Autodesk Fusion 360 part; units mm, degrees
(part 2 of 3)
  spline S292 degree 3 poles (-119.6869, 0.8689) (-119.9271, 0.6416) (-120.1494, 0.602) (-120.3986, 0.874) knots 0 0 0 0 1 1 1 1
  spline S293 degree 3 poles (-120.3986, 0.874) (-120.6491, 1.1474) (-120.9787, 1.2392) (-121.3477, 1.1905) knots 0 0 0 0 1 1 1 1
  spline S294 degree 3 poles (-121.3477, 1.1905) (-121.5549, 1.1631) (-121.713, 1.0742) (-121.7659, 0.8603) knots 0 0 0 0 1 1 1 1
  spline S295 degree 3 poles (-121.7659, 0.8603) (-121.8248, 0.6223) (-121.7241, 0.4521) (-121.5106, 0.3512) knots 0 0 0 0 1 1 1 1
  spline S296 degree 3 poles (-121.5106, 0.3512) (-121.1033, 0.1585) (-120.6785, -0.0017) (-120.2865, -0.221) knots 0 0 0 0 1 1 1 1
  spline S297 degree 3 poles (-120.2865, -0.221) (-119.417, -0.7075) (-119.0197, -1.6781) (-119.281, -2.6156) knots 0 0 0 0 1 1 1 1
  spline S298 degree 3 poles (-119.281, -2.6156) (-119.4987, -3.3967) (-120.0372, -3.8655) (-120.8096, -4.0071) knots 0 0 0 0 1 1 1 1
  spline S299 degree 3 poles (-120.8096, -4.0071) (-121.664, -4.1637) (-122.4734, -4.0633) (-123.0688, -3.3088) knots 0 0 0 0 1 1 1 1
  spline S300 degree 3 poles (-123.0688, -3.3088) (-123.2667, -3.0579) (-123.2642, -2.865) (-123.0212, -2.6394) knots 0 0 0 0 1 1 1 1
  spline S301 degree 3 poles (-123.0212, -2.6394) (-122.4403, -2.1) (-122.3298, -2.0653) (-121.6554, -2.4022) knots 0 0 0 0 1 1 1 1
  spline S302 degree 3 poles (-121.6554, -2.4022) (-121.3441, -2.5577) (-121.0624, -2.5327) (-120.8747, -2.2487) knots 0 0 0 0 1 1 1 1
  spline S303 degree 3 poles (-120.8747, -2.2487) (-120.6748, -1.9465) (-120.8812, -1.7016) (-121.122, -1.5519) knots 0 0 0 0 1 1 1 1
  spline S304 degree 3 poles (-121.122, -1.5519) (-121.3991, -1.3797) (-121.711, -1.259) (-122.0168, -1.1387) knots 0 0 0 0 1 1 1 1
  spline S305 degree 3 poles (-122.0168, -1.1387) (-122.3785, -0.9965) (-122.7031, -0.8076) (-122.9863, -0.484) knots 0 0 0 0 1 1 1 1
  spline S306 degree 3 poles (-129.5748, -3.9986) (-130.0779, -3.6151) (-129.8967, -3.1145) (-129.8126, -2.6894) knots 0 0 0 0 1 1 1 1
  spline S307 degree 3 poles (-129.8126, -2.6894) (-129.7416, -2.3309) (-129.331, -2.397) (-129.0513, -2.4282) knots 0 0 0 0 1 1 1 1
  spline S308 degree 3 poles (-129.0513, -2.4282) (-128.508, -2.4889) (-128.3687, -2.2636) (-128.3813, -1.7476) knots 0 0 0 0 1 1 1 1
  spline S309 degree 3 poles (-128.3813, -1.7476) (-128.4113, -0.5149) (-128.3747, 0.7193) (-128.3882, 1.9526) knots 0 0 0 0 1 1 1 1
  spline S310 degree 3 poles (-128.3882, 1.9526) (-128.3933, 2.4157) (-128.2265, 2.6017) (-127.7479, 2.6027) knots 0 0 0 0 1 1 1 1
  spline S311 degree 3 poles (-127.7479, 2.6027) (-126.5945, 2.6052) (-126.5944, 2.623) (-126.5928, 1.4801) knots 0 0 0 0 1 1 1 1
  spline S312 degree 3 poles (-126.5928, 1.4801) (-126.5912, 0.3682) (-126.5753, -0.7439) (-126.5959, -1.8554) knots 0 0 0 0 1 1 1 1
  spline S313 degree 3 poles (-126.5959, -1.8554) (-126.6037, -2.2776) (-126.4743, -2.4417) (-126.0346, -2.4338) knots 0 0 0 0 1 1 1 1
  spline S314 degree 3 poles (-126.0346, -2.4338) (-125.2421, -2.4195) (-124.8555, -3.1182) (-125.2315, -3.822) knots 0 0 0 0 1 1 1 1
  spline S315 degree 3 poles (-125.2315, -3.822) (-125.3441, -4.0327) (-125.5369, -4.0315) (-125.7256, -4.0311) knots 0 0 0 0 1 1 1 1
  spline S316 degree 3 poles (-125.7256, -4.0311) (-126.9936, -4.028) (-128.2615, -4.0194) (-129.5748, -3.9986) knots 0 0 0 0 1 1 1 1
  spline S317 degree 3 poles (-151.8161, -2.4591) (-151.7724, -2.7435) (-151.9201, -3.0231) (-151.6525, -3.2497) knots 0 0 0 0 1 1 1 1
  spline S318 degree 3 poles (-151.6525, -3.2497) (-151.3521, -3.0403) (-151.5054, -2.7385) (-151.4726, -2.4901) knots 0 0 0 0 1 1 1 1
  spline S319 degree 3 poles (-151.4726, -2.4901) (-151.45, -2.3191) (-151.4678, -2.1432) (-151.4568, -1.9701) knots 0 0 0 0 1 1 1 1
  spline S320 degree 3 poles (-151.4568, -1.9701) (-151.4461, -1.8001) (-151.3237, -1.7311) (-151.1748, -1.7199) knots 0 0 0 0 1 1 1 1
  spline S321 degree 3 poles (-151.1748, -1.7199) (-150.9979, -1.7065) (-150.9253, -1.8309) (-150.9167, -1.9813) knots 0 0 0 0 1 1 1 1
  spline S322 degree 3 poles (-150.9167, -1.9813) (-150.9028, -2.2236) (-150.9108, -2.467) (-150.9054, -2.7099) knots 0 0 0 0 1 1 1 1
  spline S323 degree 3 poles (-150.9054, -2.7099) (-150.8995, -2.9796) (-150.9741, -3.2813) (-150.5847, -3.3799) knots 0 0 0 0 1 1 1 1
  spline S324 degree 3 poles (-150.5847, -3.3799) (-150.4389, -3.4169) (-150.4547, -3.5703) (-150.4745, -3.6907) knots 0 0 0 0 1 1 1 1
  spline S325 degree 3 poles (-150.4745, -3.6907) (-150.4965, -3.8235) (-150.6099, -3.8351) (-150.7149, -3.8355) knots 0 0 0 0 1 1 1 1
  spline S326 degree 3 poles (-150.7149, -3.8355) (-151.2185, -3.8373) (-151.7221, -3.8387) (-152.2257, -3.833) knots 0 0 0 0 1 1 1 1
  spline S327 degree 3 poles (-152.2257, -3.833) (-152.6223, -3.8286) (-152.4677, -3.3848) (-152.687, -3.2345) knots 0 0 0 0 1 1 1 1
  spline S328 degree 3 poles (-152.687, -3.2345) (-152.7158, -3.2563) (-152.7521, -3.2703) (-152.7654, -3.296) knots 0 0 0 0 1 1 1 1
  spline S329 degree 3 poles (-152.7654, -3.296) (-152.8885, -3.5349) (-152.8614, -3.9369) (-153.3119, -3.8241) knots 0 0 0 0 1 1 1 1
  spline S330 degree 3 poles (-153.3119, -3.8241) (-153.728, -3.72) (-153.5082, -3.3696) (-153.5522, -3.1274) knots 0 0 0 0 1 1 1 1
  spline S331 degree 3 poles (-153.5522, -3.1274) (-153.5827, -2.9593) (-153.5583, -2.7811) (-153.5579, -2.6074) knots 0 0 0 0 1 1 1 1
  spline S332 degree 3 poles (-153.5579, -2.6074) (-153.5558, -1.7753) (-153.4341, -1.6381) (-152.6172, -1.747) knots 0 0 0 0 1 1 1 1
  spline S333 degree 3 poles (-152.6172, -1.747) (-152.381, -1.7784) (-152.1385, -1.7461) (-151.9071, -1.8076) knots 0 0 0 0 1 1 1 1
  spline S334 degree 3 poles (-151.9071, -1.8076) (-151.7549, -1.9976) (-151.8414, -2.2141) (-151.8161, -2.4591) knots 0 0 0 0 1 1 1 1
  line L4 (0, -35) -> (-76, -35)
  line L5 (-76, -35) -> (-76, 111)
  line L6 (-76, 111) -> (0, 111)
  line L7 (0, 111) -> (0, -35)
  circle A0 centre (-38, 38) radius 9.8923
  constraint horizontal L4
  constraint vertical L5
  constraint horizontal L6
  constraint vertical L7
  constraint coincident L0.start L3.end
  constraint coincident L1.end L2.start
move_body "Move2" bodies 1 to x (1, 0, 0) y (0, 1, 0) z (0, 0, 1) at (-97.5748, 51.7195, 0)
sketch "Sketch12" plane through (0, 0, 0) normal (0, 0, -1) x (1, 0, 0)
  spline S0 degree 3 poles (-152.6172, -1.747) (-152.381, -1.7784) (-152.1385, -1.7461) (-151.9071, -1.8076) knots 0 0 0 0 1 1 1 1
  line L0 (-152.268, -1.7658) -> (-152.3095, -2.6636)
  line L1 (-152.4767, -2.7329) -> (-152.5571, -2.6598)
  line L2 (-152.6831, -2.6528) -> (-152.8325, -2.7611)
  spline S1 degree 3 poles (-153.5579, -2.6074) (-153.5558, -1.7753) (-153.4341, -1.6381) (-152.6172, -1.747) knots 0 0 0 0 1 1 1 1
  line L3 (-152.9911, -2.6801) -> (-152.9911, -1.7147)
  arc A0 (-152.4767, -2.7329) -> (-152.3095, -2.6636) centre (-152.4094, -2.659) ccw
  arc A1 (-152.9911, -2.6801) -> (-152.8325, -2.7611) centre (-152.8911, -2.6801) ccw
  arc A2 (-152.5571, -2.6598) -> (-152.6831, -2.6528) centre (-152.6244, -2.7338) ccw
  dimension "d50" = 0.1
  constraint coincident S0 L0.start
  constraint coincident S1 L3.end
  constraint vertical L3
  constraint tangent L0 A0
  constraint tangent L1 A0
  constraint tangent L2 A1
  constraint tangent L3 A1
  constraint equal A0 A1
  constraint tangent L1 A2
  constraint tangent L2 A2
  constraint equal A0 A2
  measures "d50" radius of A0
extrude "Extrude8" cut sketch "Sketch11" against normal blind 2 contours S0 S1 S2 S3 S4 S5 S6 S7 S8 S9 S10 S11 S12 S13 S14 S15 S16 S17 S18 S19 S20 S21 S22 S23 S24 S25 S26 S27 S28 S29 S30 S31 S32 S33 S34 S35 S36 S37 S38 S39 S40 S41 S42 S43 S44 S45 S46 S47 S48 S49 S50 S51 S52 | S53 S54 S55 S56 S57 S58 S59 S60 S61 S62 S63 S64 S65 S66 S67 S68 S69 S70 S71 S72 S73 S74 S75 S76 S77 S78 S79 S80 S81 S82 S83 S84 S85 S86 S87 | S88 S89 S90 S91 S92 S93 S94 S95 S96 S97 S98 S99 S100 S101 S102 | S103 S104 S105 S106 S107 S108 S109 | S110 S111 S112 S113 S114 S115 S116 S117 S118 S119 | S132 S133 S134 S135 S136 S137 S138 S139 S140 S141 S142 S143 S144 S145 S146 S147 S148 S149 S150 S151 S152 | S160 S161 S162 S163 S164 S165 S166 S167 | S175 S176 S177 S178 S179 S180 S181 S182 S183 S184 S185 S186 S187 S188 S189 S190 S191 S192 S193 S194 | S195 S196 S197 S198 S199 S200 S201 S202 | S211 S212 S213 S214 S215 S216 S217 S218 S219 S220 S221 S222 S223 | S224 S225 S226 S227 S228 S229 S230 S231 S232 S233 S234 S235 S236 | S237 S238 S239 S240 S241 S242 S243 S244 S245 S246 S247 S248 S249 S250 S251 S252 S253 | S254 S255 S256 S257 S258 S259 S260 S261 S262 | S269 S270 S271 S272 S273 S274 S275 S276 S277 S278 S279 S280 S281 S282 | S287 S288 S289 S290 S291 S292 S293 S294 S295 S296 S297 S298 S299 S300 S301 S302 S303 S304 S305 | S306 S307 S308 S309 S310 S311 S312 S313 S314 S315 S316 | S317 S318 S319 S320 S321 S322 S323 S324 S325 S326 S327 S328 S329 S330 S331 S332 S333 S334
extrude "Extrude9" add sketch "Sketch12" against normal blind 4
sketch "Sketch10" plane through (0, 0, 0) normal (0, 0, -1) x (1, 0, 0)
  line L0 (-76, 111) -> (-76, -35)
  line L1 (-76, -35) -> (0, -35)
  line L2 (0, -35) -> (0, 111)
  line L3 (0, 111) -> (-76, 111)
  spline S0 degree 3 poles (-40.4317, 17.6006) (-39.8291, 17.28) (-39.2423, 16.9866) (-38.6763, 16.6573) knots 0 0 0 0 1 1 1 1
  spline S1 degree 3 poles (-38.6763, 16.6573) (-38.3724, 16.4806) (-38.1212, 16.4902) (-37.8148, 16.6546) knots 0 0 0 0 1 1 1 1
  spline S2 degree 3 poles (-37.8148, 16.6546) (-34.9507, 18.1923) (-32.084, 19.7253) (-29.2103, 21.245) knots 0 0 0 0 1 1 1 1
  spline S3 degree 3 poles (-29.2103, 21.245) (-25.08, 23.4292) (-20.946, 25.6063) (-16.8046, 27.7693) knots 0 0 0 0 1 1 1 1
  spline S4 degree 3 poles (-16.8046, 27.7693) (-16.4301, 27.9649) (-16.287, 28.1873) (-16.3158, 28.6025) knots 0 0 0 0 1 1 1 1
  spline S5 degree 3 poles (-16.3158, 28.6025) (-16.3521, 29.128) (-16.3245, 29.6579) (-16.3245, 30.1627) knots 0 0 0 0 1 1 1 1
  spline S6 degree 3 poles (-16.3245, 30.1627) (-16.5073, 30.2364) (-16.5975, 30.1526) (-16.6925, 30.1048) knots 0 0 0 0 1 1 1 1
  spline S7 degree 3 poles (-16.6925, 30.1048) (-20.6237, 28.1267) (-24.5543, 26.1475) (-28.4844, 24.1672) knots 0 0 0 0 1 1 1 1
  spline S8 degree 3 poles (-28.4844, 24.1672) (-30.3499, 23.2272) (-32.2141, 22.2846) (-34.0792, 21.3436) knots 0 0 0 0 1 1 1 1
  spline S9 degree 3 poles (-34.0792, 21.3436) (-34.1453, 21.3102) (-34.2127, 21.2786) (-34.2814, 21.251) knots 0 0 0 0 1 1 1 1
  spline S10 degree 3 poles (-34.2814, 21.251) (-34.4117, 21.1986) (-34.5493, 21.1531) (-34.6489, 21.2964) knots 0 0 0 0 1 1 1 1
  spline S11 degree 3 poles (-34.6489, 21.2964) (-34.7335, 21.4181) (-34.6738, 21.5343) (-34.5964, 21.6372) knots 0 0 0 0 1 1 1 1
  spline S12 degree 3 poles (-34.5964, 21.6372) (-34.314, 22.0126) (-34.0358, 22.3915) (-33.7448, 22.7602) knots 0 0 0 0 1 1 1 1
  spline S13 degree 3 poles (-33.7448, 22.7602) (-32.7338, 24.0411) (-31.6965, 25.3003) (-30.6356, 26.5404) knots 0 0 0 0 1 1 1 1
  spline S14 degree 3 poles (-30.6356, 26.5404) (-30.4816, 26.7204) (-30.3529, 26.738) (-30.1615, 26.6279) knots 0 0 0 0 1 1 1 1
  spline S15 degree 3 poles (-30.1615, 26.6279) (-29.7972, 26.4184) (-29.4194, 26.2318) (-29.0606, 26.0138) knots 0 0 0 0 1 1 1 1
  spline S16 degree 3 poles (-29.0606, 26.0138) (-28.8311, 25.8744) (-28.6558, 25.8728) (-28.4311, 26.0438) knots 0 0 0 0 1 1 1 1
  spline S17 degree 3 poles (-28.4311, 26.0438) (-26.8276, 27.2638) (-25.2138, 28.4704) (-23.6035, 29.6815) knots 0 0 0 0 1 1 1 1
  spline S18 degree 3 poles (-23.6035, 29.6815) (-22.4773, 30.5286) (-21.3445, 31.3672) (-20.2289, 32.228) knots 0 0 0 0 1 1 1 1
  spline S19 degree 3 poles (-20.2289, 32.228) (-19.8034, 32.5564) (-19.3869, 32.7208) (-18.8147, 32.6999) knots 0 0 0 0 1 1 1 1
  spline S20 degree 3 poles (-18.8147, 32.6999) (-17.2091, 32.6411) (-15.6, 32.6802) (-13.9922, 32.6803) knots 0 0 0 0 1 1 1 1
  spline S21 degree 3 poles (-13.9922, 32.6803) (-13.4089, 32.6804) (-13.4081, 32.6799) (-13.408, 32.0922) knots 0 0 0 0 1 1 1 1
  spline S22 degree 3 poles (-13.408, 32.0922) (-13.4074, 30.2495) (-13.4144, 28.4068) (-13.4008, 26.5642) knots 0 0 0 0 1 1 1 1
  spline S23 degree 3 poles (-13.4008, 26.5642) (-13.3985, 26.2517) (-13.4942, 26.0732) (-13.7752, 25.926) knots 0 0 0 0 1 1 1 1
  spline S24 degree 3 poles (-13.7752, 25.926) (-17.0053, 24.2335) (-20.2295, 22.5294) (-23.4551, 20.828) knots 0 0 0 0 1 1 1 1
  spline S25 degree 3 poles (-23.4551, 20.828) (-26.9757, 18.971) (-30.4947, 17.1109) (-34.0173, 15.2576) knots 0 0 0 0 1 1 1 1
  spline S26 degree 3 poles (-34.0173, 15.2576) (-35.3082, 14.5785) (-36.6107, 13.9215) (-37.8999, 13.2394) knots 0 0 0 0 1 1 1 1
  spline S27 degree 3 poles (-37.8999, 13.2394) (-38.1595, 13.102) (-38.3656, 13.1055) (-38.6238, 13.2425) knots 0 0 0 0 1 1 1 1
  spline S28 degree 3 poles (-38.6238, 13.2425) (-42.249, 15.1663) (-45.8792, 17.0807) (-49.508, 18.9978) knots 0 0 0 0 1 1 1 1
  spline S29 degree 3 poles (-49.508, 18.9978) (-53.2898, 20.9957) (-57.0716, 22.9936) (-60.853, 24.9924) knots 0 0 0 0 1 1 1 1
  spline S30 degree 3 poles (-60.853, 24.9924) (-61.465, 25.3159) (-62.0712, 25.6507) (-62.6872, 25.9664) knots 0 0 0 0 1 1 1 1
  spline S31 degree 3 poles (-62.6872, 25.9664) (-62.9254, 26.0885) (-63.0226, 26.2507) (-63.0215, 26.5222) knots 0 0 0 0 1 1 1 1
  spline S32 degree 3 poles (-63.0215, 26.5222) (-63.0144, 28.4514) (-63.0143, 30.3807) (-63.0276, 32.3099) knots 0 0 0 0 1 1 1 1
  spline S33 degree 3 poles (-63.0276, 32.3099) (-63.0297, 32.6276) (-62.8983, 32.7181) (-62.6112, 32.7178) knots 0 0 0 0 1 1 1 1
  spline S34 degree 3 poles (-62.6112, 32.7178) (-59.2844, 32.7145) (-55.9577, 32.7158) (-52.6309, 32.7162) knots 0 0 0 0 1 1 1 1
  spline S35 degree 3 poles (-52.6309, 32.7162) (-52.4544, 32.7162) (-52.2888, 32.6722) (-52.1287, 32.6012) knots 0 0 0 0 1 1 1 1
  spline S36 degree 3 poles (-52.1287, 32.6012) (-51.835, 32.4709) (-51.5523, 32.2943) (-51.245, 32.2198) knots 0 0 0 0 1 1 1 1
  spline S37 degree 3 poles (-51.245, 32.2198) (-50.2747, 31.9847) (-49.8666, 31.2768) (-49.5459, 30.4169) knots 0 0 0 0 1 1 1 1
  spline S38 degree 3 poles (-49.5459, 30.4169) (-49.0582, 29.1093) (-48.5003, 27.8279) (-47.9695, 26.5365) knots 0 0 0 0 1 1 1 1
  spline S39 degree 3 poles (-47.9695, 26.5365) (-47.7908, 26.1019) (-47.7698, 26.092) (-47.3574, 26.3088) knots 0 0 0 0 1 1 1 1
  spline S40 degree 3 poles (-47.3574, 26.3088) (-47.0185, 26.487) (-46.6822, 26.6723) (-46.3573, 26.8746) knots 0 0 0 0 1 1 1 1
  spline S41 degree 3 poles (-46.3573, 26.8746) (-46.1633, 26.9955) (-46.0404, 26.9885) (-45.8926, 26.7975) knots 0 0 0 0 1 1 1 1
  spline S42 degree 3 poles (-45.8926, 26.7975) (-44.6895, 25.2429) (-43.4747, 23.6974) (-42.2713, 22.1432) knots 0 0 0 0 1 1 1 1
  spline S43 degree 3 poles (-42.2713, 22.1432) (-42.0708, 21.8842) (-41.8458, 21.6294) (-41.7841, 21.2734) knots 0 0 0 0 1 1 1 1
  spline S44 degree 3 poles (-41.7841, 21.2734) (-42.0555, 21.1046) (-42.2709, 21.2649) (-42.4785, 21.3719) knots 0 0 0 0 1 1 1 1
  spline S45 degree 3 poles (-42.4785, 21.3719) (-43.7858, 22.0462) (-45.0845, 22.7375) (-46.3942, 23.4072) knots 0 0 0 0 1 1 1 1
  spline S46 degree 3 poles (-46.3942, 23.4072) (-48.6832, 24.5777) (-50.9766, 25.7399) (-53.2712, 26.8996) knots 0 0 0 0 1 1 1 1
  spline S47 degree 3 poles (-53.2712, 26.8996) (-55.4005, 27.9757) (-57.5337, 29.0441) (-59.6655, 30.1154) knots 0 0 0 0 1 1 1 1
  spline S48 degree 3 poles (-59.6655, 30.1154) (-59.7749, 30.1704) (-59.8863, 30.2215) (-60.0223, 30.2865) knots 0 0 0 0 1 1 1 1
  spline S49 degree 3 poles (-60.0223, 30.2865) (-60.1404, 29.9708) (-60.0305, 29.6583) (-60.088, 29.3669) knots 0 0 0 0 1 1 1 1
  spline S50 degree 3 poles (-60.088, 29.3669) (-60.2909, 28.3392) (-59.8047, 27.8515) (-58.9038, 27.3866) knots 0 0 0 0 1 1 1 1
  spline S51 degree 3 poles (-58.9038, 27.3866) (-54.1257, 24.9209) (-49.3893, 22.3743) (-44.64, 19.8529) knots 0 0 0 0 1 1 1 1
  spline S52 degree 3 poles (-44.64, 19.8529) (-43.2428, 19.1111) (-41.8507, 18.3598) (-40.4317, 17.6006) knots 0 0 0 0 1 1 1 1
  spline S53 degree 3 poles (-60.7731, 44.8042) (-61.379, 44.8028) (-61.9479, 44.8068) (-62.5166, 44.7979) knots 0 0 0 0 1 1 1 1
  spline S54 degree 3 poles (-62.5166, 44.7979) (-62.8551, 44.7926) (-63.0169, 44.9347) (-63.0161, 45.283) knots 0 0 0 0 1 1 1 1
  spline S55 degree 3 poles (-63.0161, 45.283) (-63.0126, 46.7669) (-63.0135, 48.2508) (-63.0232, 49.7346) knots 0 0 0 0 1 1 1 1
  spline S56 degree 3 poles (-63.0232, 49.7346) (-63.0249, 49.9964) (-62.8688, 50.1007) (-62.6743, 50.2018) knots 0 0 0 0 1 1 1 1
  spline S57 degree 3 poles (-62.6743, 50.2018) (-59.1547, 52.032) (-55.6309, 53.8543) (-52.1182, 55.6976) knots 0 0 0 0 1 1 1 1
  spline S58 degree 3 poles (-52.1182, 55.6976) (-47.6092, 58.0637) (-43.1082, 60.4449) (-38.6081, 62.8278) knots 0 0 0 0 1 1 1 1
  spline S59 degree 3 poles (-38.6081, 62.8278) (-38.3627, 62.9578) (-38.1752, 62.9654) (-37.925, 62.8346) knots 0 0 0 0 1 1 1 1
  spline S60 degree 3 poles (-37.925, 62.8346) (-31.9, 59.6869) (-25.8711, 56.547) (-19.8417, 53.4079) knots 0 0 0 0 1 1 1 1
  spline S61 degree 3 poles (-19.8417, 53.4079) (-17.8246, 52.3578) (-15.8067, 51.3093) (-13.7828, 50.2726) knots 0 0 0 0 1 1 1 1
  spline S62 degree 3 poles (-13.7828, 50.2726) (-13.5161, 50.136) (-13.4027, 49.9747) (-13.4054, 49.6715) knots 0 0 0 0 1 1 1 1
  spline S63 degree 3 poles (-13.4054, 49.6715) (-13.4177, 48.2372) (-13.409, 46.8027) (-13.4115, 45.3683) knots 0 0 0 0 1 1 1 1
  spline S64 degree 3 poles (-13.4115, 45.3683) (-13.4123, 44.9361) (-13.5267, 44.8077) (-13.9596, 44.8067) knots 0 0 0 0 1 1 1 1
  spline S65 degree 3 poles (-13.9596, 44.8067) (-17.0015, 44.8001) (-20.0435, 44.7985) (-23.0854, 44.8015) knots 0 0 0 0 1 1 1 1
  spline S66 degree 3 poles (-23.0854, 44.8015) (-23.5349, 44.8019) (-23.5738, 44.8812) (-23.5723, 45.3313) knots 0 0 0 0 1 1 1 1
  spline S67 degree 3 poles (-23.5723, 45.3313) (-23.5683, 46.5055) (-23.5838, 47.6797) (-23.5895, 48.8539) knots 0 0 0 0 1 1 1 1
  spline S68 degree 3 poles (-23.5895, 48.8539) (-23.5902, 48.9871) (-23.6153, 49.1267) (-23.506, 49.2698) knots 0 0 0 0 1 1 1 1
  spline S69 degree 3 poles (-23.506, 49.2698) (-23.298, 49.2853) (-23.1263, 49.153) (-22.9473, 49.06) knots 0 0 0 0 1 1 1 1
  spline S70 degree 3 poles (-22.9473, 49.06) (-21.6969, 48.4105) (-20.4452, 47.7632) (-19.2035, 47.0975) knots 0 0 0 0 1 1 1 1
  spline S71 degree 3 poles (-19.2035, 47.0975) (-18.8987, 46.9341) (-18.6443, 46.9303) (-18.3398, 47.0966) knots 0 0 0 0 1 1 1 1
  spline S72 degree 3 poles (-18.3398, 47.0966) (-17.725, 47.4322) (-17.0917, 47.734) (-16.427, 48.0695) knots 0 0 0 0 1 1 1 1
  spline S73 degree 3 poles (-16.427, 48.0695) (-16.639, 48.2716) (-16.8651, 48.37) (-17.0785, 48.4809) knots 0 0 0 0 1 1 1 1
  spline S74 degree 3 poles (-17.0785, 48.4809) (-21.6512, 50.8586) (-26.2286, 53.2273) (-30.7981, 55.611) knots 0 0 0 0 1 1 1 1
  spline S75 degree 3 poles (-30.7981, 55.611) (-33.1871, 56.8572) (-35.5642, 58.1262) (-37.9424, 59.3928) knots 0 0 0 0 1 1 1 1
  spline S76 degree 3 poles (-37.9424, 59.3928) (-38.1605, 59.509) (-38.3305, 59.5209) (-38.5568, 59.4007) knots 0 0 0 0 1 1 1 1
  spline S77 degree 3 poles (-38.5568, 59.4007) (-44.092, 56.4629) (-49.6152, 53.5023) (-55.1866, 50.6331) knots 0 0 0 0 1 1 1 1
  spline S78 degree 3 poles (-55.1866, 50.6331) (-56.7251, 49.8408) (-58.2575, 49.0368) (-59.7922, 48.2373) knots 0 0 0 0 1 1 1 1
  spline S79 degree 3 poles (-59.7922, 48.2373) (-59.8673, 48.1982) (-59.9376, 48.1502) (-60.0614, 48.0753) knots 0 0 0 0 1 1 1 1
  spline S80 degree 3 poles (-60.0614, 48.0753) (-59.2865, 47.6875) (-58.553, 47.319) (-57.8182, 46.9534) knots 0 0 0 0 1 1 1 1
  spline S81 degree 3 poles (-57.8182, 46.9534) (-57.6304, 46.86) (-57.4853, 46.988) (-57.336, 47.0659) knots 0 0 0 0 1 1 1 1
  spline S82 degree 3 poles (-57.336, 47.0659) (-56.12, 47.701) (-54.9066, 48.3411) (-53.6895, 48.9741) knots 0 0 0 0 1 1 1 1
  spline S83 degree 3 poles (-53.6895, 48.9741) (-53.463, 49.0919) (-53.2411, 49.2297) (-52.9865, 49.2697) knots 0 0 0 0 1 1 1 1
  spline S84 degree 3 poles (-52.9865, 49.2697) (-52.8438, 49.1569) (-52.8848, 49.0106) (-52.8844, 48.8826) knots 0 0 0 0 1 1 1 1
  spline S85 degree 3 poles (-52.8844, 48.8826) (-52.8809, 47.6708) (-52.895, 46.4588) (-52.8757, 45.2472) knots 0 0 0 0 1 1 1 1
  spline S86 degree 3 poles (-52.8757, 45.2472) (-52.8697, 44.876) (-53.0127, 44.7914) (-53.354, 44.7932) knots 0 0 0 0 1 1 1 1
  spline S87 degree 3 poles (-53.354, 44.7932) (-55.8146, 44.8058) (-58.2753, 44.8024) (-60.7731, 44.8042) knots 0 0 0 0 1 1 1 1
  spline S88 degree 3 poles (-33.9538, 25.8681) (-35.2112, 24.3401) (-36.4457, 22.8276) (-37.6952, 21.3276) knots 0 0 0 0 1 1 1 1
  spline S89 degree 3 poles (-37.6952, 21.3276) (-38.2233, 20.6936) (-38.3279, 20.7041) (-38.8426, 21.3321) knots 0 0 0 0 1 1 1 1
  spline S90 degree 3 poles (-38.8426, 21.3321) (-41.3725, 24.4188) (-43.9003, 27.5072) (-46.4306, 30.5935) knots 0 0 0 0 1 1 1 1
  spline S91 degree 3 poles (-46.4306, 30.5935) (-46.8928, 31.1572) (-47.3652, 31.7126) (-47.8282, 32.2757) knots 0 0 0 0 1 1 1 1
  spline S92 degree 3 poles (-47.8282, 32.2757) (-47.9118, 32.3775) (-48.0221, 32.4689) (-48.0433, 32.7114) knots 0 0 0 0 1 1 1 1
  spline S93 degree 3 poles (-48.0433, 32.7114) (-47.6374, 32.7114) (-47.2384, 32.7149) (-46.8394, 32.7106) knots 0 0 0 0 1 1 1 1
  spline S94 degree 3 poles (-46.8394, 32.7106) (-46.1352, 32.7031) (-45.431, 32.6806) (-44.7269, 32.6858) knots 0 0 0 0 1 1 1 1
  spline S95 degree 3 poles (-44.7269, 32.6858) (-44.4673, 32.6878) (-44.2812, 32.596) (-44.1119, 32.4122) knots 0 0 0 0 1 1 1 1
  spline S96 degree 3 poles (-44.1119, 32.4122) (-42.2788, 30.4217) (-40.4423, 28.4342) (-38.6078, 26.4449) knots 0 0 0 0 1 1 1 1
  spline S97 degree 3 poles (-38.6078, 26.4449) (-38.3108, 26.1228) (-38.2997, 26.1207) (-37.989, 26.4557) knots 0 0 0 0 1 1 1 1
  spline S98 degree 3 poles (-37.989, 26.4557) (-36.1322, 28.4573) (-34.2746, 30.4583) (-32.4196, 32.4616) knots 0 0 0 0 1 1 1 1
  spline S99 degree 3 poles (-32.4196, 32.4616) (-32.2783, 32.6142) (-32.1252, 32.7157) (-31.9081, 32.7153) knots 0 0 0 0 1 1 1 1
  spline S100 degree 3 poles (-31.9081, 32.7153) (-30.8452, 32.7133) (-29.7822, 32.7167) (-28.7192, 32.7158) knots 0 0 0 0 1 1 1 1
  spline S101 degree 3 poles (-28.7192, 32.7158) (-28.623, 32.7158) (-28.5179, 32.728) (-28.4106, 32.5827) knots 0 0 0 0 1 1 1 1
  spline S102 degree 3 poles (-28.4106, 32.5827) (-30.2462, 30.3592) (-32.0915, 28.124) (-33.9538, 25.8681) knots 0 0 0 0 1 1 1 1
  spline S103 degree 3 poles (-36.6568, 52.1406) (-40.0754, 52.1405) (-43.4569, 52.1405) (-46.8398, 52.1405) knots 0 0 0 0 1 1 1 1
  spline S104 degree 3 poles (-46.8398, 52.1405) (-46.8608, 52.3819) (-46.6993, 52.4122) (-46.5935, 52.4723) knots 0 0 0 0 1 1 1 1
  spline S105 degree 3 poles (-46.5935, 52.4723) (-43.9617, 53.9679) (-41.2947, 55.3988) (-38.6189, 56.8136) knots 0 0 0 0 1 1 1 1
  spline S106 degree 3 poles (-38.6189, 56.8136) (-38.3374, 56.9625) (-38.1122, 56.9581) (-37.8283, 56.8058) knots 0 0 0 0 1 1 1 1
  spline S107 degree 3 poles (-37.8283, 56.8058) (-35.1719, 55.3813) (-32.5073, 53.9721) (-29.8465, 52.5558) knots 0 0 0 0 1 1 1 1
  spline S108 degree 3 poles (-29.8465, 52.5558) (-29.7104, 52.4833) (-29.5438, 52.4342) (-29.4755, 52.1406) knots 0 0 0 0 1 1 1 1
  spline S109 degree 3 poles (-29.4755, 52.1406) (-31.876, 52.1406) (-34.2479, 52.1406) (-36.6568, 52.1406) knots 0 0 0 0 1 1 1 1
  spline S110 degree 3 poles (-20.8539, 41.4702) (-20.3904, 42.1319) (-19.775, 42.4135) (-18.997, 42.3986) knots 0 0 0 0 1 1 1 1
  spline S111 degree 3 poles (-18.997, 42.3986) (-18.0949, 42.3813) (-17.192, 42.3826) (-16.2899, 42.4001) knots 0 0 0 0 1 1 1 1
  spline S112 degree 3 poles (-16.2899, 42.4001) (-15.9623, 42.4064) (-15.8634, 42.2913) (-15.8655, 41.9707) knots 0 0 0 0 1 1 1 1
  spline S113 degree 3 poles (-15.8655, 41.9707) (-15.8796, 39.8075) (-15.8777, 37.6442) (-15.8823, 35.481) knots 0 0 0 0 1 1 1 1
  spline S114 degree 3 poles (-15.8823, 35.481) (-15.8828, 35.2853) (-15.8483, 35.0565) (-16.1592, 35.0713) knots 0 0 0 0 1 1 1 1
  spline S115 degree 3 poles (-16.1592, 35.0713) (-17.2827, 35.125) (-18.406, 34.9465) (-19.5294, 35.0716) knots 0 0 0 0 1 1 1 1
  spline S116 degree 3 poles (-19.5294, 35.0716) (-20.5103, 35.1808) (-21.3536, 36.3249) (-21.2111, 37.3017) knots 0 0 0 0 1 1 1 1
  spline S117 degree 3 poles (-21.2111, 37.3017) (-21.1416, 37.7784) (-21.0196, 38.2217) (-20.7196, 38.5973) knots 0 0 0 0 1 1 1 1
  spline S118 degree 3 poles (-20.7196, 38.5973) (-20.5782, 38.7743) (-20.6677, 38.8854) (-20.765, 39.0183) knots 0 0 0 0 1 1 1 1
  spline S119 degree 3 poles (-20.765, 39.0183) (-21.3407, 39.8044) (-21.3351, 40.6163) (-20.8539, 41.4702) knots 0 0 0 0 1 1 1 1
  spline S120 degree 3 poles (-18.5026, 38.1201) (-18.5886, 38.1195) (-18.675, 38.1234) (-18.7606, 38.1176) knots 0 0 0 0 1 1 1 1
  spline S121 degree 3 poles (-18.7606, 38.1176) (-19.2119, 38.0874) (-19.4978, 37.7917) (-19.495, 37.361) knots 0 0 0 0 1 1 1 1
  spline S122 degree 3 poles (-19.495, 37.361) (-19.4924, 36.9517) (-19.2114, 36.7005) (-18.7391, 36.6887) knots 0 0 0 0 1 1 1 1
  spline S123 degree 3 poles (-18.7391, 36.6887) (-18.5794, 36.6848) (-18.4196, 36.6867) (-18.2598, 36.6866) knots 0 0 0 0 1 1 1 1
  spline S124 degree 3 poles (-18.2598, 36.6866) (-17.6908, 36.686) (-17.6908, 36.6861) (-17.6532, 37.2637) knots 0 0 0 0 1 1 1 1
  spline S125 degree 3 poles (-17.6532, 37.2637) (-17.5975, 38.1183) (-17.5975, 38.1183) (-18.5026, 38.1201) knots 0 0 0 0 1 1 1 1
  spline S126 degree 3 poles (-19.4871, 40.2977) (-19.4722, 39.8404) (-19.2908, 39.6494) (-18.8441, 39.6251) knots 0 0 0 0 1 1 1 1
  spline S127 degree 3 poles (-18.8441, 39.6251) (-18.5741, 39.6104) (-18.304, 39.5968) (-18.0337, 39.5882) knots 0 0 0 0 1 1 1 1
  spline S128 degree 3 poles (-18.0337, 39.5882) (-17.8027, 39.5808) (-17.6578, 39.6641) (-17.6651, 39.929) knots 0 0 0 0 1 1 1 1
  spline S129 degree 3 poles (-17.6651, 39.929) (-17.6929, 40.9305) (-17.4648, 40.8355) (-18.5413, 40.8515) knots 0 0 0 0 1 1 1 1
  spline S130 degree 3 poles (-18.5413, 40.8515) (-18.6028, 40.8524) (-18.6649, 40.8573) (-18.7258, 40.8512) knots 0 0 0 0 1 1 1 1
  spline S131 degree 3 poles (-18.7258, 40.8512) (-19.0635, 40.8173) (-19.3466, 40.6989) (-19.4871, 40.2977) knots 0 0 0 0 1 1 1 1
  spline S132 degree 3 poles (-54.9627, 37.5472) (-54.963, 36.8183) (-54.9713, 36.1263) (-54.9595, 35.4346) knots 0 0 0 0 1 1 1 1
  spline S133 degree 3 poles (-54.9595, 35.4346) (-54.9549, 35.163) (-55.057, 35.0621) (-55.3269, 35.0646) knots 0 0 0 0 1 1 1 1
  spline S134 degree 3 poles (-55.3269, 35.0646) (-56.2287, 35.073) (-57.1309, 35.0525) (-58.0324, 35.0691) knots 0 0 0 0 1 1 1 1
  spline S135 degree 3 poles (-58.0324, 35.0691) (-59.0976, 35.0888) (-60.0624, 36.0814) (-60.1353, 37.1478) knots 0 0 0 0 1 1 1 1
  spline S136 degree 3 poles (-60.1353, 37.1478) (-60.2035, 38.1432) (-59.9756, 38.9854) (-59.0855, 39.5482) knots 0 0 0 0 1 1 1 1
  spline S137 degree 3 poles (-59.0855, 39.5482) (-58.9438, 39.6378) (-58.9557, 39.7431) (-59.0258, 39.8624) knots 0 0 0 0 1 1 1 1
  spline S138 degree 3 poles (-59.0258, 39.8624) (-59.0884, 39.9688) (-59.1783, 40.0632) (-59.2213, 40.1762) knots 0 0 0 0 1 1 1 1
  spline S139 degree 3 poles (-59.2213, 40.1762) (-59.4187, 40.6946) (-59.7898, 40.8791) (-60.3224, 40.781) knots 0 0 0 0 1 1 1 1
  spline S140 degree 3 poles (-60.3224, 40.781) (-60.6487, 40.7209) (-60.7709, 40.8532) (-60.739, 41.1861) knots 0 0 0 0 1 1 1 1
  spline S141 degree 3 poles (-60.739, 41.1861) (-60.7109, 41.4801) (-60.7236, 41.7787) (-60.73, 42.0751) knots 0 0 0 0 1 1 1 1
  spline S142 degree 3 poles (-60.73, 42.0751) (-60.7345, 42.2811) (-60.638, 42.3703) (-60.4419, 42.3688) knots 0 0 0 0 1 1 1 1
  spline S143 degree 3 poles (-60.4419, 42.3688) (-60.0591, 42.3661) (-59.6763, 42.3667) (-59.2937, 42.3573) knots 0 0 0 0 1 1 1 1
  spline S144 degree 3 poles (-59.2937, 42.3573) (-58.7406, 42.3438) (-58.4337, 41.9734) (-58.1717, 41.5545) knots 0 0 0 0 1 1 1 1
  spline S145 degree 3 poles (-58.1717, 41.5545) (-57.9032, 41.1253) (-57.6415, 40.6914) (-57.3911, 40.2514) knots 0 0 0 0 1 1 1 1
  spline S146 degree 3 poles (-57.3911, 40.2514) (-57.2646, 40.029) (-57.0832, 39.9713) (-56.8614, 40.0334) knots 0 0 0 0 1 1 1 1
  spline S147 degree 3 poles (-56.8614, 40.0334) (-56.6402, 40.0954) (-56.7227, 40.2971) (-56.7195, 40.443) knots 0 0 0 0 1 1 1 1
  spline S148 degree 3 poles (-56.7195, 40.443) (-56.7093, 40.9246) (-56.715, 41.4066) (-56.7134, 41.8884) knots 0 0 0 0 1 1 1 1
  spline S149 degree 3 poles (-56.7134, 41.8884) (-56.7118, 42.3704) (-56.7074, 42.3746) (-56.2081, 42.3776) knots 0 0 0 0 1 1 1 1
  spline S150 degree 3 poles (-56.2081, 42.3776) (-55.9487, 42.3792) (-55.6878, 42.3612) (-55.4301, 42.3824) knots 0 0 0 0 1 1 1 1
  spline S151 degree 3 poles (-55.4301, 42.3824) (-55.0792, 42.4112) (-54.9532, 42.2823) (-54.9572, 41.9208) knots 0 0 0 0 1 1 1 1
  spline S152 degree 3 poles (-54.9572, 41.9208) (-54.9733, 40.4755) (-54.9632, 39.0299) (-54.9627, 37.5472) knots 0 0 0 0 1 1 1 1
  spline S153 degree 3 poles (-58.0444, 38.2874) (-58.3511, 38.0656) (-58.5698, 37.7886) (-58.4902, 37.3881) knots 0 0 0 0 1 1 1 1
  spline S154 degree 3 poles (-58.4902, 37.3881) (-58.4117, 36.9932) (-58.1221, 36.7136) (-57.7764, 36.6849) knots 0 0 0 0 1 1 1 1
  spline S155 degree 3 poles (-57.7764, 36.6849) (-57.5072, 36.6626) (-57.235, 36.6783) (-56.9642, 36.6761) knots 0 0 0 0 1 1 1 1
  spline S156 degree 3 poles (-56.9642, 36.6761) (-56.797, 36.6748) (-56.7164, 36.7538) (-56.7174, 36.9236) knots 0 0 0 0 1 1 1 1
  spline S157 degree 3 poles (-56.7174, 36.9236) (-56.7198, 37.3423) (-56.7181, 37.761) (-56.7184, 38.1798) knots 0 0 0 0 1 1 1 1
  spline S158 degree 3 poles (-56.7184, 38.1798) (-56.7184, 38.3052) (-56.7625, 38.4079) (-56.9033, 38.4052) knots 0 0 0 0 1 1 1 1
  spline S159 degree 3 poles (-56.9033, 38.4052) (-57.2689, 38.3984) (-57.643, 38.485) (-58.0444, 38.2874) knots 0 0 0 0 1 1 1 1
  spline S160 degree 3 poles (-23.874, 42.1871) (-23.0228, 41.712) (-22.5919, 41.0229) (-22.6061, 40.0609) knots 0 0 0 0 1 1 1 1
  spline S161 degree 3 poles (-22.6061, 40.0609) (-22.6186, 39.2082) (-22.6151, 38.3552) (-22.608, 37.5024) knots 0 0 0 0 1 1 1 1
  spline S162 degree 3 poles (-22.608, 37.5024) (-22.5931, 35.7153) (-23.9133, 34.7055) (-25.7287, 34.96) knots 0 0 0 0 1 1 1 1
  spline S163 degree 3 poles (-25.7287, 34.96) (-26.7675, 35.1056) (-27.4548, 35.6911) (-27.7891, 36.6894) knots 0 0 0 0 1 1 1 1
  spline S164 degree 3 poles (-27.7891, 36.6894) (-27.8456, 36.858) (-27.8508, 37.0283) (-27.8504, 37.2014) knots 0 0 0 0 1 1 1 1
  spline S165 degree 3 poles (-27.8504, 37.2014) (-27.848, 38.1408) (-27.8442, 39.0802) (-27.8439, 40.0196) knots 0 0 0 0 1 1 1 1
  spline S166 degree 3 poles (-27.8439, 40.0196) (-27.8435, 41.2536) (-27.0562, 42.2202) (-25.8313, 42.3729) knots 0 0 0 0 1 1 1 1
  spline S167 degree 3 poles (-25.8313, 42.3729) (-25.1903, 42.4528) (-24.5217, 42.4946) (-23.874, 42.1871) knots 0 0 0 0 1 1 1 1
  spline S168 degree 3 poles (-24.9384, 40.7719) (-25.589, 40.9512) (-26.033, 40.6223) (-26.0453, 39.959) knots 0 0 0 0 1 1 1 1
  spline S169 degree 3 poles (-26.0453, 39.959) (-26.0542, 39.4775) (-26.0828, 38.9962) (-26.0852, 38.5147) knots 0 0 0 0 1 1 1 1
  spline S170 degree 3 poles (-26.0852, 38.5147) (-26.0874, 38.0709) (-26.1294, 37.6246) (-26.0394, 37.1837) knots 0 0 0 0 1 1 1 1
  spline S171 degree 3 poles (-26.0394, 37.1837) (-25.9569, 36.7798) (-25.6197, 36.5712) (-25.1034, 36.603) knots 0 0 0 0 1 1 1 1
  spline S172 degree 3 poles (-25.1034, 36.603) (-24.7203, 36.6265) (-24.4362, 36.8762) (-24.4298, 37.2552) knots 0 0 0 0 1 1 1 1
  spline S173 degree 3 poles (-24.4298, 37.2552) (-24.4137, 38.2064) (-24.4185, 39.1581) (-24.421, 40.1095) knots 0 0 0 0 1 1 1 1
  spline S174 degree 3 poles (-24.421, 40.1095) (-24.4218, 40.4289) (-24.5814, 40.6459) (-24.9384, 40.7719) knots 0 0 0 0 1 1 1 1
  spline S175 degree 3 poles (-52.9583, 42.3725) (-51.4771, 42.3748) (-50.0307, 42.3713) (-48.5843, 42.3784) knots 0 0 0 0 1 1 1 1
  spline S176 degree 3 poles (-48.5843, 42.3784) (-48.3258, 42.3797) (-48.2024, 42.3083) (-48.2031, 42.023) knots 0 0 0 0 1 1 1 1
  spline S177 degree 3 poles (-48.2031, 42.023) (-48.2082, 39.8353) (-48.2074, 37.6475) (-48.1942, 35.4598) knots 0 0 0 0 1 1 1 1
  spline S178 degree 3 poles (-48.1942, 35.4598) (-48.1923, 35.1447) (-48.3094, 35.0609) (-48.6055, 35.0633) knots 0 0 0 0 1 1 1 1
  spline S179 degree 3 poles (-48.6055, 35.0633) (-50.0148, 35.0746) (-51.4242, 35.0739) (-52.8334, 35.0653) knots 0 0 0 0 1 1 1 1
  spline S180 degree 3 poles (-52.8334, 35.0653) (-53.1172, 35.0636) (-53.2306, 35.1571) (-53.2251, 35.4505) knots 0 0 0 0 1 1 1 1
  spline S181 degree 3 poles (-53.2251, 35.4505) (-53.1975, 36.9401) (-53.4094, 36.6563) (-52.0333, 36.6804) knots 0 0 0 0 1 1 1 1
  spline S182 degree 3 poles (-52.0333, 36.6804) (-51.3445, 36.6925) (-50.6552, 36.6825) (-49.9642, 36.6825) knots 0 0 0 0 1 1 1 1
  spline S183 degree 3 poles (-49.9642, 36.6825) (-49.876, 37.0429) (-49.8992, 37.3634) (-49.8985, 37.6821) knots 0 0 0 0 1 1 1 1
  spline S184 degree 3 poles (-49.8985, 37.6821) (-49.898, 37.9372) (-50.0798, 37.9376) (-50.2595, 37.9393) knots 0 0 0 0 1 1 1 1
  spline S185 degree 3 poles (-50.2595, 37.9393) (-51.0996, 37.9475) (-51.9399, 37.9697) (-52.7797, 37.9559) knots 0 0 0 0 1 1 1 1
  spline S186 degree 3 poles (-52.7797, 37.9559) (-53.1111, 37.9505) (-53.2076, 38.0701) (-53.2033, 38.3848) knots 0 0 0 0 1 1 1 1
  spline S187 degree 3 poles (-53.2033, 38.3848) (-53.1851, 39.7212) (-53.3283, 39.4761) (-52.1129, 39.4964) knots 0 0 0 0 1 1 1 1
  spline S188 degree 3 poles (-52.1129, 39.4964) (-51.495, 39.5067) (-50.8766, 39.5064) (-50.2587, 39.4946) knots 0 0 0 0 1 1 1 1
  spline S189 degree 3 poles (-50.2587, 39.4946) (-49.9897, 39.4895) (-49.8817, 39.5832) (-49.889, 39.8604) knots 0 0 0 0 1 1 1 1
  spline S190 degree 3 poles (-49.889, 39.8604) (-49.9186, 40.9702) (-49.725, 40.7722) (-50.7939, 40.788) knots 0 0 0 0 1 1 1 1
  spline S191 degree 3 poles (-50.7939, 40.788) (-51.4737, 40.7981) (-52.1539, 40.7986) (-52.8336, 40.7859) knots 0 0 0 0 1 1 1 1
  spline S192 degree 3 poles (-52.8336, 40.7859) (-53.1168, 40.7806) (-53.2442, 40.8748) (-53.2276, 41.17) knots 0 0 0 0 1 1 1 1
  spline S193 degree 3 poles (-53.2276, 41.17) (-53.2109, 41.4658) (-53.2224, 41.7632) (-53.2234, 42.0599) knots 0 0 0 0 1 1 1 1
  spline S194 degree 3 poles (-53.2234, 42.0599) (-53.2239, 42.222) (-53.1952, 42.3597) (-52.9583, 42.3725) knots 0 0 0 0 1 1 1 1
  spline S195 degree 3 poles (-42.1556, 42.3809) (-41.6033, 42.372) (-41.602, 42.372) (-41.6018, 41.8713) knots 0 0 0 0 1 1 1 1
  spline S196 degree 3 poles (-41.6018, 41.8713) (-41.6011, 39.7588) (-41.6081, 37.6463) (-41.5944, 35.5339) knots 0 0 0 0 1 1 1 1
  spline S197 degree 3 poles (-41.5944, 35.5339) (-41.5921, 35.1877) (-41.6792, 35.0544) (-42.0469, 35.0657) knots 0 0 0 0 1 1 1 1
  spline S198 degree 3 poles (-42.0469, 35.0657) (-42.8614, 35.0908) (-43.6773, 35.0693) (-44.4926, 35.0747) knots 0 0 0 0 1 1 1 1
  spline S199 degree 3 poles (-44.4926, 35.0747) (-45.5808, 35.0819) (-46.4712, 35.9686) (-46.4768, 37.0531) knots 0 0 0 0 1 1 1 1
  spline S200 degree 3 poles (-46.4768, 37.0531) (-46.4824, 38.1278) (-46.4325, 39.2051) (-46.4921, 40.2766) knots 0 0 0 0 1 1 1 1
  spline S201 degree 3 poles (-46.4921, 40.2766) (-46.5442, 41.2123) (-45.5948, 42.3769) (-44.3412, 42.3859) knots 0 0 0 0 1 1 1 1
  spline S202 degree 3 poles (-44.3412, 42.3859) (-43.6247, 42.391) (-42.9082, 42.3831) (-42.1556, 42.3809) knots 0 0 0 0 1 1 1 1
  spline S203 degree 3 poles (-44.7949, 38.1045) (-44.7948, 37.8825) (-44.7953, 37.6605) (-44.7945, 37.4384) knots 0 0 0 0 1 1 1 1
  spline S204 degree 3 poles (-44.7945, 37.4384) (-44.7923, 36.8612) (-44.6274, 36.6924) (-44.0521, 36.6797) knots 0 0 0 0 1 1 1 1
  spline S205 degree 3 poles (-44.0521, 36.6797) (-43.9288, 36.6769) (-43.8043, 36.6888) (-43.6822, 36.6761) knots 0 0 0 0 1 1 1 1
  spline S206 degree 3 poles (-43.6822, 36.6761) (-43.3742, 36.6442) (-43.2723, 36.7783) (-43.2764, 37.0818) knots 0 0 0 0 1 1 1 1
  spline S207 degree 3 poles (-43.2764, 37.0818) (-43.2893, 38.0437) (-43.2715, 39.006) (-43.2818, 39.968) knots 0 0 0 0 1 1 1 1
  spline S208 degree 3 poles (-43.2818, 39.968) (-43.2918, 40.8989) (-43.1024, 40.7917) (-44.1392, 40.7847) knots 0 0 0 0 1 1 1 1
  spline S209 degree 3 poles (-44.1392, 40.7847) (-44.5582, 40.7819) (-44.7914, 40.5247) (-44.7946, 40.1026) knots 0 0 0 0 1 1 1 1
  spline S210 degree 3 poles (-44.7946, 40.1026) (-44.7994, 39.4613) (-44.7953, 38.8198) (-44.7949, 38.1045) knots 0 0 0 0 1 1 1 1
  spline S211 degree 3 poles (-32.6992, 35.9174) (-32.6994, 35.0721) (-32.6994, 35.0721) (-33.5061, 35.0544) knots 0 0 0 0 1 1 1 1
  spline S212 degree 3 poles (-33.5061, 35.0544) (-34.3825, 35.0351) (-34.3824, 35.0351) (-34.3824, 35.922) knots 0 0 0 0 1 1 1 1
  spline S213 degree 3 poles (-34.3824, 35.922) (-34.3824, 37.3442) (-34.3826, 38.7663) (-34.3825, 40.1884) knots 0 0 0 0 1 1 1 1
  spline S214 degree 3 poles (-34.3825, 40.1884) (-34.3825, 41.5002) (-33.5563, 42.373) (-32.2396, 42.4525) knots 0 0 0 0 1 1 1 1
  spline S215 degree 3 poles (-32.2396, 42.4525) (-31.4556, 42.4998) (-30.7425, 42.335) (-30.1557, 41.7723) knots 0 0 0 0 1 1 1 1
  spline S216 degree 3 poles (-30.1557, 41.7723) (-29.7427, 41.3763) (-29.5125, 40.9002) (-29.5111, 40.3262) knots 0 0 0 0 1 1 1 1
  spline S217 degree 3 poles (-29.5111, 40.3262) (-29.5073, 38.7186) (-29.5186, 37.1108) (-29.5022, 35.5034) knots 0 0 0 0 1 1 1 1
  spline S218 degree 3 poles (-29.5022, 35.5034) (-29.4988, 35.1665) (-29.6122, 35.0524) (-29.9382, 35.0319) knots 0 0 0 0 1 1 1 1
  spline S219 degree 3 poles (-29.9382, 35.0319) (-31.1917, 34.9531) (-31.1909, 34.9453) (-31.1913, 36.1877) knots 0 0 0 0 1 1 1 1
  spline S220 degree 3 poles (-31.1913, 36.1877) (-31.1917, 37.4985) (-31.1863, 38.8093) (-31.1967, 40.1201) knots 0 0 0 0 1 1 1 1
  spline S221 degree 3 poles (-31.1967, 40.1201) (-31.2014, 40.711) (-31.8079, 41.0563) (-32.3351, 40.7847) knots 0 0 0 0 1 1 1 1
  spline S222 degree 3 poles (-32.3351, 40.7847) (-32.626, 40.6349) (-32.7015, 40.3787) (-32.7005, 40.0719) knots 0 0 0 0 1 1 1 1
  spline S223 degree 3 poles (-32.7005, 40.0719) (-32.6962, 38.6992) (-32.699, 37.3266) (-32.6992, 35.9174) knots 0 0 0 0 1 1 1 1
  spline S224 degree 3 poles (-36.2013, 40.367) (-36.2026, 38.7355) (-36.2138, 37.1411) (-36.198, 35.5469) knots 0 0 0 0 1 1 1 1
  spline S225 degree 3 poles (-36.198, 35.5469) (-36.1943, 35.1753) (-36.3041, 35.0275) (-36.683, 35.0624) knots 0 0 0 0 1 1 1 1
  spline S226 degree 3 poles (-36.683, 35.0624) (-36.9269, 35.0849) (-37.1768, 35.0581) (-37.4227, 35.0376) knots 0 0 0 0 1 1 1 1
  spline S227 degree 3 poles (-37.4227, 35.0376) (-37.7457, 35.0106) (-37.8821, 35.1126) (-37.8782, 35.471) knots 0 0 0 0 1 1 1 1
  spline S228 degree 3 poles (-37.8782, 35.471) (-37.8606, 37.1022) (-37.8778, 38.7338) (-37.865, 40.3651) knots 0 0 0 0 1 1 1 1
  spline S229 degree 3 poles (-37.865, 40.3651) (-37.8625, 40.682) (-37.9472, 40.8142) (-38.2817, 40.7963) knots 0 0 0 0 1 1 1 1
  spline S230 degree 3 poles (-38.2817, 40.7963) (-38.7253, 40.7726) (-39.1715, 40.8) (-39.6161, 40.7873) knots 0 0 0 0 1 1 1 1
  spline S231 degree 3 poles (-39.6161, 40.7873) (-39.8941, 40.7794) (-40.0336, 40.8721) (-40.018, 41.1691) knots 0 0 0 0 1 1 1 1
  spline S232 degree 3 poles (-40.018, 41.1691) (-40.0039, 41.4403) (-40.0033, 41.7134) (-40.0172, 41.9846) knots 0 0 0 0 1 1 1 1
  spline S233 degree 3 poles (-40.0172, 41.9846) (-40.0321, 42.2776) (-39.8967, 42.378) (-39.6188, 42.3761) knots 0 0 0 0 1 1 1 1
  spline S234 degree 3 poles (-39.6188, 42.3761) (-38.6054, 42.3689) (-37.5919, 42.3688) (-36.5784, 42.3735) knots 0 0 0 0 1 1 1 1
  spline S235 degree 3 poles (-36.5784, 42.3735) (-36.3142, 42.3747) (-36.196, 42.2688) (-36.2004, 41.9984) knots 0 0 0 0 1 1 1 1
  spline S236 degree 3 poles (-36.2004, 41.9984) (-36.209, 41.4671) (-36.202, 40.9356) (-36.2013, 40.367) knots 0 0 0 0 1 1 1 1
  spline S237 degree 3 poles (-43.3577, 45.6465) (-43.3582, 46.8058) (-43.3641, 47.9294) (-43.3541, 49.0529) knots 0 0 0 0 1 1 1 1
  spline S238 degree 3 poles (-43.3541, 49.0529) (-43.3522, 49.266) (-43.4681, 49.5477) (-43.1425, 49.6508) knots 0 0 0 0 1 1 1 1
  spline S239 degree 3 poles (-43.1425, 49.6508) (-42.7653, 49.7701) (-42.3164, 49.659) (-42.1418, 49.3917) knots 0 0 0 0 1 1 1 1
  spline S240 degree 3 poles (-42.1418, 49.3917) (-41.8718, 48.9786) (-41.6165, 48.556) (-41.353, 48.1386) knots 0 0 0 0 1 1 1 1
  spline S241 degree 3 poles (-41.353, 48.1386) (-41.3022, 48.0583) (-41.2422, 47.9837) (-41.1134, 47.9177) knots 0 0 0 0 1 1 1 1
  spline S242 degree 3 poles (-41.1134, 47.9177) (-41.1134, 48.3302) (-41.1179, 48.7428) (-41.1122, 49.1552) knots 0 0 0 0 1 1 1 1
  spline S243 degree 3 poles (-41.1122, 49.1552) (-41.1059, 49.613) (-41.0509, 49.664) (-40.598, 49.6691) knots 0 0 0 0 1 1 1 1
  spline S244 degree 3 poles (-40.598, 49.6691) (-40.4869, 49.6703) (-40.3756, 49.6642) (-40.2647, 49.6695) knots 0 0 0 0 1 1 1 1
  spline S245 degree 3 poles (-40.2647, 49.6695) (-40.0376, 49.6803) (-39.9108, 49.5816) (-39.9101, 49.3487) knots 0 0 0 0 1 1 1 1
  spline S246 degree 3 poles (-39.9101, 49.3487) (-39.906, 48.003) (-39.9037, 46.6572) (-39.9006, 45.3114) knots 0 0 0 0 1 1 1 1
  spline S247 degree 3 poles (-39.9006, 45.3114) (-39.9002, 45.1396) (-39.9734, 45.0275) (-40.1518, 45.0031) knots 0 0 0 0 1 1 1 1
  spline S248 degree 3 poles (-40.1518, 45.0031) (-40.4476, 44.9627) (-40.7469, 44.9027) (-40.943, 45.2273) knots 0 0 0 0 1 1 1 1
  spline S249 degree 3 poles (-40.943, 45.2273) (-41.2431, 45.7237) (-41.5487, 46.2168) (-41.8522, 46.7111) knots 0 0 0 0 1 1 1 1
  spline S250 degree 3 poles (-41.8522, 46.7111) (-41.9229, 46.8262) (-41.9948, 46.9406) (-42.142, 47.0511) knots 0 0 0 0 1 1 1 1
  spline S251 degree 3 poles (-42.142, 47.0511) (-42.142, 46.5678) (-42.1417, 46.0846) (-42.142, 45.6013) knots 0 0 0 0 1 1 1 1
  spline S252 degree 3 poles (-42.142, 45.6013) (-42.1425, 45.019) (-42.1913, 44.9617) (-42.6855, 44.961) knots 0 0 0 0 1 1 1 1
  spline S253 degree 3 poles (-42.6855, 44.961) (-43.2759, 44.9602) (-43.3504, 45.0322) (-43.3577, 45.6465) knots 0 0 0 0 1 1 1 1
  spline S254 degree 3 poles (-47.5021, 49.4429) (-47.1215, 49.7041) (-46.7103, 49.7039) (-46.3028, 49.7039) knots 0 0 0 0 1 1 1 1
  spline S255 degree 3 poles (-46.3028, 49.7039) (-45.9695, 49.7039) (-45.6363, 49.6751) (-45.3031, 49.675) knots 0 0 0 0 1 1 1 1
  spline S256 degree 3 poles (-45.3031, 49.675) (-45.0578, 49.675) (-44.9402, 49.5809) (-44.9409, 49.3251) knots 0 0 0 0 1 1 1 1
  spline S257 degree 3 poles (-44.9409, 49.3251) (-44.9444, 47.9906) (-44.9442, 46.6561) (-44.9374, 45.3217) knots 0 0 0 0 1 1 1 1
  spline S258 degree 3 poles (-44.9374, 45.3217) (-44.9361, 45.0678) (-45.049, 44.9584) (-45.2909, 44.9586) knots 0 0 0 0 1 1 1 1
  spline S259 degree 3 poles (-45.2909, 44.9586) (-45.7851, 44.9591) (-46.281, 44.9347) (-46.7731, 44.9671) knots 0 0 0 0 1 1 1 1
  spline S260 degree 3 poles (-46.7731, 44.9671) (-47.5469, 45.0181) (-48.0793, 45.6107) (-48.1036, 46.437) knots 0 0 0 0 1 1 1 1
  spline S261 degree 3 poles (-48.1036, 46.437) (-48.1229, 47.0913) (-48.1141, 47.7468) (-48.1054, 48.4015) knots 0 0 0 0 1 1 1 1
  spline S262 degree 3 poles (-48.1054, 48.4015) (-48.0995, 48.844) (-47.8602, 49.166) (-47.5021, 49.4429) knots 0 0 0 0 1 1 1 1
  spline S263 degree 3 poles (-46.5271, 48.6392) (-46.736, 48.5889) (-46.9198, 48.4696) (-46.9275, 48.2555) knots 0 0 0 0 1 1 1 1
  spline S264 degree 3 poles (-46.9275, 48.2555) (-46.9491, 47.6522) (-46.9618, 47.0456) (-46.921, 46.4442) knots 0 0 0 0 1 1 1 1
  spline S265 degree 3 poles (-46.921, 46.4442) (-46.901, 46.1486) (-46.6264, 46.0903) (-46.3536, 46.1024) knots 0 0 0 0 1 1 1 1
  spline S266 degree 3 poles (-46.3536, 46.1024) (-46.0701, 46.1149) (-46.0975, 46.3156) (-46.0967, 46.4996) knots 0 0 0 0 1 1 1 1
  spline S267 degree 3 poles (-46.0967, 46.4996) (-46.0943, 47.0795) (-46.1036, 47.6596) (-46.0914, 48.2393) knots 0 0 0 0 1 1 1 1
  spline S268 degree 3 poles (-46.0914, 48.2393) (-46.0856, 48.5159) (-46.1762, 48.6665) (-46.5271, 48.6392) knots 0 0 0 0 1 1 1 1
  spline S269 degree 3 poles (-35.4639, 47.3502) (-35.6647, 46.6577) (-35.8443, 45.9908) (-35.9757, 45.3118) knots 0 0 0 0 1 1 1 1
  spline S270 degree 3 poles (-35.9757, 45.3118) (-35.9873, 45.2517) (-35.9918, 45.1718) (-36.0312, 45.1382) knots 0 0 0 0 1 1 1 1
  spline S271 degree 3 poles (-36.0312, 45.1382) (-36.3949, 44.8278) (-36.8323, 45.0204) (-37.2356, 44.9765) knots 0 0 0 0 1 1 1 1
  spline S272 degree 3 poles (-37.2356, 44.9765) (-37.4465, 44.9535) (-37.5332, 45.1009) (-37.5813, 45.2891) knots 0 0 0 0 1 1 1 1
  spline S273 degree 3 poles (-37.5813, 45.2891) (-37.9167, 46.6035) (-38.2647, 47.9148) (-38.5909, 49.2315) knots 0 0 0 0 1 1 1 1
  spline S274 degree 3 poles (-38.5909, 49.2315) (-38.693, 49.6438) (-38.6067, 49.7241) (-38.1754, 49.7423) knots 0 0 0 0 1 1 1 1
  spline S275 degree 3 poles (-38.1754, 49.7423) (-38.1014, 49.7454) (-38.0239, 49.7397) (-37.9543, 49.7598) knots 0 0 0 0 1 1 1 1
  spline S276 degree 3 poles (-37.9543, 49.7598) (-37.6281, 49.8544) (-37.4658, 49.7104) (-37.3947, 49.4026) knots 0 0 0 0 1 1 1 1
  spline S277 degree 3 poles (-37.3947, 49.4026) (-37.3549, 49.2304) (-37.3883, 48.985) (-37.1655, 48.9394) knots 0 0 0 0 1 1 1 1
  spline S278 degree 3 poles (-37.1655, 48.9394) (-36.8897, 48.883) (-36.5933, 48.8807) (-36.3215, 48.9614) knots 0 0 0 0 1 1 1 1
  spline S279 degree 3 poles (-36.3215, 48.9614) (-36.1727, 49.0056) (-36.181, 49.2063) (-36.1387, 49.3462) knots 0 0 0 0 1 1 1 1
  spline S280 degree 3 poles (-36.1387, 49.3462) (-36.0337, 49.6932) (-35.2585, 49.9094) (-34.9988, 49.6584) knots 0 0 0 0 1 1 1 1
  spline S281 degree 3 poles (-34.9988, 49.6584) (-34.875, 49.5388) (-34.9213, 49.3798) (-34.9582, 49.2386) knots 0 0 0 0 1 1 1 1
  spline S282 degree 3 poles (-34.9582, 49.2386) (-35.1202, 48.6177) (-35.2886, 47.9985) (-35.4639, 47.3502) knots 0 0 0 0 1 1 1 1
  spline S283 degree 3 poles (-36.8942, 47.3563) (-36.839, 47.2399) (-36.8548, 47.0919) (-36.7206, 46.9842) knots 0 0 0 0 1 1 1 1
  spline S284 degree 3 poles (-36.7206, 46.9842) (-36.6614, 47.2632) (-36.5601, 47.5189) (-36.5921, 47.7978) knots 0 0 0 0 1 1 1 1
  spline S285 degree 3 poles (-36.5921, 47.7978) (-36.7236, 47.8488) (-36.8374, 47.8678) (-36.9556, 47.76) knots 0 0 0 0 1 1 1 1
  spline S286 degree 3 poles (-36.9556, 47.76) (-36.9419, 47.6472) (-36.9273, 47.5276) (-36.8942, 47.3563) knots 0 0 0 0 1 1 1 1
  spline S287 degree 3 poles (-29.2574, 47.4787) (-29.663, 48.0635) (-29.669, 48.6374) (-29.2707, 49.1871) knots 0 0 0 0 1 1 1 1
  spline S288 degree 3 poles (-29.2707, 49.1871) (-28.8317, 49.7929) (-28.1852, 49.8059) (-27.5295, 49.709) knots 0 0 0 0 1 1 1 1
  spline S289 degree 3 poles (-27.5295, 49.709) (-27.1685, 49.6556) (-26.8599, 49.4701) (-26.5938, 49.2164) knots 0 0 0 0 1 1 1 1
  spline S290 degree 3 poles (-26.5938, 49.2164) (-26.4269, 49.0573) (-26.4138, 48.9025) (-26.5834, 48.7416) knots 0 0 0 0 1 1 1 1
  spline S291 degree 3 poles (-26.5834, 48.7416) (-26.6908, 48.6397) (-26.803, 48.5428) (-26.9105, 48.441) knots 0 0 0 0 1 1 1 1
  spline S292 degree 3 poles (-26.9105, 48.441) (-27.0813, 48.2793) (-27.2394, 48.2512) (-27.4167, 48.4447) knots 0 0 0 0 1 1 1 1
  spline S293 degree 3 poles (-27.4167, 48.4447) (-27.5949, 48.6391) (-27.8294, 48.7045) (-28.0918, 48.6698) knots 0 0 0 0 1 1 1 1
  spline S294 degree 3 poles (-28.0918, 48.6698) (-28.2392, 48.6503) (-28.3517, 48.5871) (-28.3893, 48.435) knots 0 0 0 0 1 1 1 1
  spline S295 degree 3 poles (-28.3893, 48.435) (-28.4312, 48.2656) (-28.3596, 48.1446) (-28.2077, 48.0728) knots 0 0 0 0 1 1 1 1
  spline S296 degree 3 poles (-28.2077, 48.0728) (-27.918, 47.9357) (-27.6158, 47.8218) (-27.3369, 47.6657) knots 0 0 0 0 1 1 1 1
  spline S297 degree 3 poles (-27.3369, 47.6657) (-26.7185, 47.3197) (-26.4359, 46.6293) (-26.6217, 45.9624) knots 0 0 0 0 1 1 1 1
  spline S298 degree 3 poles (-26.6217, 45.9624) (-26.7766, 45.4068) (-27.1596, 45.0733) (-27.7091, 44.9726) knots 0 0 0 0 1 1 1 1
  spline S299 degree 3 poles (-27.7091, 44.9726) (-28.3168, 44.8612) (-28.8926, 44.9326) (-29.3161, 45.4694) knots 0 0 0 0 1 1 1 1
  spline S300 degree 3 poles (-29.3161, 45.4694) (-29.4569, 45.6478) (-29.4551, 45.785) (-29.2822, 45.9455) knots 0 0 0 0 1 1 1 1
  spline S301 degree 3 poles (-29.2822, 45.9455) (-28.869, 46.3292) (-28.7904, 46.3538) (-28.3107, 46.1142) knots 0 0 0 0 1 1 1 1
  spline S302 degree 3 poles (-28.3107, 46.1142) (-28.0892, 46.0036) (-27.8889, 46.0214) (-27.7553, 46.2234) knots 0 0 0 0 1 1 1 1
  spline S303 degree 3 poles (-27.7553, 46.2234) (-27.6132, 46.4384) (-27.76, 46.6125) (-27.9313, 46.7191) knots 0 0 0 0 1 1 1 1
  spline S304 degree 3 poles (-27.9313, 46.7191) (-28.1284, 46.8416) (-28.3503, 46.9274) (-28.5678, 47.0129) knots 0 0 0 0 1 1 1 1
  spline S305 degree 3 poles (-28.5678, 47.0129) (-28.825, 47.1141) (-29.0559, 47.2485) (-29.2574, 47.4787) knots 0 0 0 0 1 1 1 1
  spline S306 degree 3 poles (-33.944, 44.9787) (-34.3018, 45.2514) (-34.173, 45.6075) (-34.1131, 45.9099) knots 0 0 0 0 1 1 1 1
  spline S307 degree 3 poles (-34.1131, 45.9099) (-34.0626, 46.1649) (-33.7706, 46.1179) (-33.5716, 46.0957) knots 0 0 0 0 1 1 1 1
  spline S308 degree 3 poles (-33.5716, 46.0957) (-33.1852, 46.0526) (-33.0861, 46.2128) (-33.095, 46.5799) knots 0 0 0 0 1 1 1 1
  spline S309 degree 3 poles (-33.095, 46.5799) (-33.1164, 47.4567) (-33.0903, 48.3346) (-33.1, 49.2119) knots 0 0 0 0 1 1 1 1
  spline S310 degree 3 poles (-33.1, 49.2119) (-33.1036, 49.5413) (-32.9849, 49.6736) (-32.6445, 49.6744) knots 0 0 0 0 1 1 1 1
  spline S311 degree 3 poles (-32.6445, 49.6744) (-31.824, 49.6761) (-31.824, 49.6888) (-31.8228, 48.8758) knots 0 0 0 0 1 1 1 1
  spline S312 degree 3 poles (-31.8228, 48.8758) (-31.8217, 48.0849) (-31.8104, 47.2938) (-31.825, 46.5032) knots 0 0 0 0 1 1 1 1
  spline S313 degree 3 poles (-31.825, 46.5032) (-31.8305, 46.2029) (-31.7385, 46.0861) (-31.4258, 46.0917) knots 0 0 0 0 1 1 1 1